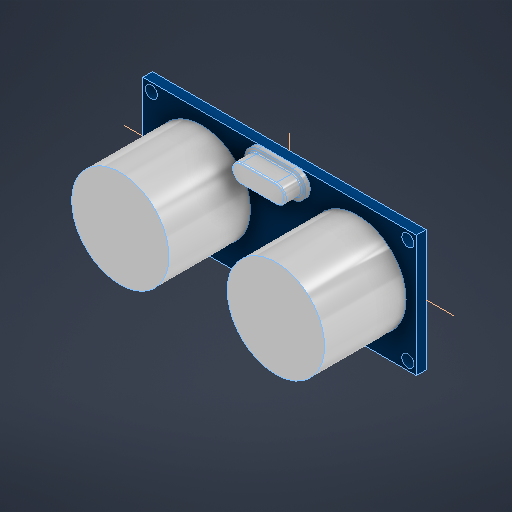
# Autodesk Inventor part: ultrasonic-sensor-2-group2
Saved by Autodesk Inventor 2026.2 (Build 302298010, 298A)
## iProperties
Created: 2026-02-24
Part Number: ultrasonic-sensor-2-group2
Material: Generic
Document SubType Name: Modeling
Designer: ts2104
Density: 1 g/cm^3
Appearance: Default
Author: ts2104
Autodesk Inventor part; units mm, degrees
ref_plane "YZ Plane" through (0, 0, 0) normal (1, 0, 0) x (0, 1, 0)
sketch "Sketch1" plane through (0, 0, 0) normal (0, 0, 1) x (1, 0, 0)
  line L0 (-22.5, 10) -> (22.5, 10)
  line L1 (22.5, 10) -> (22.5, -10)
  line L2 (22.5, -10) -> (-22.5, -10)
  line L3 (-22.5, -10) -> (-22.5, 10)
  line L4 (-22.5, 10) -> (22.5, -10) construction
  line L5 (22.5, 10) -> (-22.5, -10) construction
  line L6 (-31.5, 0) -> (31.5, 0) projected
  line L7 (0, -14) -> (0, 14) projected
  circle A0 centre (-12.8, 0) radius 8
  circle A1 centre (-21.1, -8.6) radius 1
  circle A2 centre (-21.1, 8.6) radius 1
  circle A3 centre (12.8, 0) radius 8
  circle A4 centre (21.1, -8.6) radius 1
  circle A5 centre (21.1, 8.6) radius 1
  line L8 (-5.08, -6.96) -> (5.08, -6.96)
  line L9 (5.08, -6.96) -> (5.08, -9.5)
  line L10 (5.08, -9.5) -> (-5.08, -9.5)
  line L11 (-5.08, -9.5) -> (-5.08, -6.96)
  line L12 (-5.08, -6.96) -> (5.08, -9.5) construction
  line L13 (5.08, -6.96) -> (-5.08, -9.5) construction
  line L14 (-4.13, -7.91) -> (-3.49, -7.91)
  line L15 (-3.49, -7.91) -> (-3.49, -8.55)
  line L16 (-3.49, -8.55) -> (-4.13, -8.55)
  line L17 (-4.13, -8.55) -> (-4.13, -7.91)
  line L18 (-4.13, -7.91) -> (-3.49, -8.55) construction
  line L19 (-3.49, -7.91) -> (-4.13, -8.55) construction
  line L20 (-5.08, -8.23) -> (5.08, -8.23)
  line L21 (-0.95, -7.91) -> (-1.59, -8.55) construction
  line L22 (-1.59, -7.91) -> (-0.95, -8.55) construction
  line L23 (-0.95, -8.55) -> (-1.59, -8.55)
  line L24 (-1.59, -7.91) -> (-0.95, -7.91)
  line L25 (-0.95, -7.91) -> (-0.95, -8.55)
  line L26 (-1.59, -8.55) -> (-1.59, -7.91)
  line L27 (1.59, -7.91) -> (0.95, -8.55) construction
  line L28 (0.95, -7.91) -> (1.59, -8.55) construction
  line L29 (1.59, -8.55) -> (0.95, -8.55)
  line L30 (0.95, -7.91) -> (1.59, -7.91)
  line L31 (1.59, -7.91) -> (1.59, -8.55)
  line L32 (0.95, -8.55) -> (0.95, -7.91)
  line L33 (4.13, -7.91) -> (3.49, -8.55) construction
  line L34 (3.49, -7.91) -> (4.13, -8.55) construction
  line L35 (4.13, -8.55) -> (3.49, -8.55)
  line L36 (3.49, -7.91) -> (4.13, -7.91)
  line L37 (4.13, -7.91) -> (4.13, -8.55)
  line L38 (3.49, -8.55) -> (3.49, -7.91)
  line L39 (-2.85, 10) -> (2.85, 10)
  line L40 (2.85, 10) -> (2.85, 5.6)
  line L41 (2.85, 5.6) -> (-2.85, 5.6)
  line L42 (-2.85, 5.6) -> (-2.85, 10)
  line L43 (-2.85, 10) -> (2.85, 5.6) construction
  line L44 (2.85, 10) -> (-2.85, 5.6) construction
  circle A6 centre (-2.85, 7.8) radius 2.2
  circle A7 centre (2.85, 7.8) radius 2.2
  circle A8 centre (-2.85, 7.8) radius 1.55
  line L45 (-2.85, 9.35) -> (2.85, 9.35)
  line L46 (2.85, 9.35) -> (2.85, 6.25)
  line L47 (2.85, 6.25) -> (-2.85, 6.25)
  line L48 (-2.85, 6.25) -> (-2.85, 9.35)
  line L49 (-2.85, 9.35) -> (2.85, 6.25) construction
  line L50 (2.85, 9.35) -> (-2.85, 6.25) construction
  circle A9 centre (2.85, 7.8) radius 1.55
  point P0 (0, 0)
  point P1 (0, -8.23)
  point P2 (-3.81, -8.23)
  point P3 (-1.27, -8.23)
  point P4 (1.27, -8.23)
  point P5 (3.81, -8.23)
  point P6 (0, 7.8)
  point P7 (2.85, 9.35)
  point P8 (-2.85, 6.25)
  dimension "d0" = 45
  dimension "d1" = 20
  dimension "d3" = 16
  dimension "d4" = 1.4
  dimension "d5" = 1.4
  dimension "d9" = 2
  dimension "d10" = 10.16
  dimension "d11" = 2.54
  dimension "d12" = 0.5
  dimension "d13" = 0.64
  dimension "d15" = 1.27
  dimension "d18" = 2.54
  dimension "d46" = 12.8
  dimension "d47" = 4.4
  dimension "d49" = 5.7
  dimension "d52" = 3.1
  constraints: 98 end point, 13 midpoint, 10 parallel, 8 centre point, 6 horizontal, 6 perpendicular, 6 symmetric about line, 5 point on line, 1 coincident, 1 collinear, 47 other
  measures "d0" distance of L0.start L0.end
  measures "d1" distance of L2.end L0.start
  measures "d3" diameter of A0
  measures "d4" distance from line of L3 A1.centre
  measures "d5" distance from line of A1.centre L2
  measures "d9" diameter of A1
  measures "d10" distance of L9.end L10.end
  measures "d11" distance between parallel lines of L10 L8
  measures "d12" distance between parallel lines of L2 L10
  measures "d13" distance of L16.end L14.start
  measures "d15" distance from line of L11 point (-3.81, -8.23)
  measures "d18" distance of L14.end L21.start
  measures "d46" distance from line of L7 A0.centre
  measures "d47" distance of L39.end L40.end
  measures "d49" distance of L39.start L39.end
  measures "d52" distance between parallel lines of L47 L45
extrude "Extrusion1" add sketch "Sketch1" along normal blind 1.6 contours L0 A6 L41 L7 L6 A0 L3 | A6 L45 L42 | L42 A8 A6 | L0 L7 L45 A6 | L6 A0 L7 L8 L11 L10 L2 L3 | L0 A7 L45 L7 | A8 L42 | L45 A6 L47 A8 | L42 A8 | A6 L47 L7 L41 | L42 L47 A6 | L45 L7 L47 A6 | A0 L6 | L6 A0 | A7 L40 A9 | L0 L1 L6 A3 L7 L41 A7 | L40 L45 A7 | L45 A7 L47 L7 | L7 L47 A7 L41 | L7 L10 L9 L8 L6 A3 L1 L2 | A9 L40 | A9 L47 A7 L45 | L40 A9 | A7 L47 L40 | L10 L11 L20 L17 L16 L15 L26 L23 L25 L7 | L7 L20 L32 L29 L31 L38 L35 L37 L9 L10 | A3 L6 | L6 A3 | L8 L9 L20 L37 L36 L38 L31 L30 L32 L7 | L7 L20 L25 L24 L26 L15 L14 L17 L11 L8
extrude "Extrusion2" add sketch "Sketch1" along normal blind 15 contours A0 L6 | L6 A0 | A3 L6 | L6 A3
extrude "Extrusion3" add sketch "Sketch1" against normal blind 2.4 contours L10 L11 L20 L17 L16 L15 L26 L23 L25 L7 | L7 L20 L32 L29 L31 L38 L35 L37 L9 L10 | L8 L9 L20 L37 L36 L38 L31 L30 L32 L7 | L7 L20 L25 L24 L26 L15 L14 L17 L11 L8
extrude "Extrusion4" add sketch "Sketch1" along normal blind 3 and the other way blind 3.4 separate body contours L25 L23 L26 L20 | L20 L26 L24 L25 | L32 L30 L31 L20 | L20 L31 L29 L32 | L37 L35 L38 L20 | L20 L38 L36 L37 | L20 L15 L16 L17 | L17 L14 L15 L20
sketch "Sketch2" plane through (0, 0, -3.4) normal (0, 0, -1) x (-1, 0, 0)
  line L0 (-4.13, -7.91) -> (-4.13, -8.55) projected
  line L1 (-4.13, -8.55) -> (-3.49, -8.55) projected
  line L2 (-3.49, -8.55) -> (-3.49, -7.91) projected
  line L3 (-3.49, -7.91) -> (-4.13, -7.91) projected
  line L4 (-1.59, -7.91) -> (-1.59, -8.55) projected
  line L5 (-1.59, -8.55) -> (-0.95, -8.55) projected
  line L6 (-0.95, -8.55) -> (-0.95, -7.91) projected
  line L7 (-0.95, -7.91) -> (-1.59, -7.91) projected
  line L8 (0.95, -7.91) -> (0.95, -8.55) projected
  line L9 (0.95, -8.55) -> (1.59, -8.55) projected
  line L10 (1.59, -8.55) -> (1.59, -7.91) projected
  line L11 (1.59, -7.91) -> (0.95, -7.91) projected
  line L12 (3.49, -7.91) -> (3.49, -8.55) projected
  line L13 (3.49, -8.55) -> (4.13, -8.55) projected
  line L14 (4.13, -8.55) -> (4.13, -7.91) projected
  line L15 (4.13, -7.91) -> (3.49, -7.91) projected
  point P0 (0, 0)
revolve "Revolution1" add sketch "Sketch2" angle 90 about axis through (4.13, -8.55, -3.4) along (-1, 0, 0) bodies 2
sketch "Sketch3" plane through (0.95, -8.55, 3) normal (0, -1, 0) x (1, 0, 0)
  line L0 (0, -6.4) -> (0.64, -6.4) projected
  line L1 (2.54, -6.4) -> (3.18, -6.4) projected
  line L2 (-2.54, -6.4) -> (-1.9, -6.4) projected
  line L3 (-5.08, -6.4) -> (-4.44, -6.4) projected
  line L4 (-5.08, -7.04) -> (-5.08, 0) projected
  line L5 (-5.08, -7.04) -> (-4.44, -7.04)
  line L6 (-4.44, -7.04) -> (-4.44, -6.4)
  line L7 (-4.44, -6.4) -> (-5.08, -6.4)
  line L8 (-5.08, -6.4) -> (-5.08, -7.04)
  line L9 (-2.54, -7.04) -> (-1.9, -7.04)
  line L10 (-1.9, -7.04) -> (-1.9, -6.4)
  line L11 (-1.9, -6.4) -> (-2.54, -6.4)
  line L12 (-2.54, -6.4) -> (-2.54, -7.04)
  line L13 (0, -7.04) -> (0.64, -7.04)
  line L14 (0.64, -7.04) -> (0.64, -6.4)
  line L15 (0.64, -6.4) -> (0, -6.4)
  line L16 (0, -6.4) -> (0, -7.04)
  line L17 (2.54, -7.04) -> (3.18, -7.04)
  line L18 (3.18, -7.04) -> (3.18, -6.4)
  line L19 (3.18, -6.4) -> (2.54, -6.4)
  line L20 (2.54, -6.4) -> (2.54, -7.04)
  point P0 (-0.95, -3)
  dimension "d36" = 2.54
  constraints: 32 end point, 2 horizontal, 2 parallel, 1 perpendicular, 27 other
  measures "d36" distance of L3.start point (-2.54, -6.4)
extrude "Extrusion5" add sketch "Sketch3" along normal blind 6 separate body
sketch "Sketch4" plane through (0, 0, 1.6) normal (0, 0, 1) x (1, 0, 0)
  circle A0 centre (-12.8, 0) radius 8 projected
  circle A1 centre (12.8, 0) radius 8 projected
  point P0 (0, 0)
combine bodies "Combine1" operation type add bodies to combine 3 2
ref_plane "Work Plane1" through (0, 0, 1.6) normal (0, 0, 1) x (1, 0, 0)
split body "Split1" result two bodies by plane through (0, 0, 1.6) normal (0, 0, 1) bodies 1 first body at (-5.3971, 1.2031, 6.0667) (20.2029, 1.2031, 6.0667)
fillet "Fillet1" radius 0.2 4 edges at (-3.81, -8.55, -3.4) (-1.27, -8.55, -3.4) (1.27, -8.55, -3.4) (3.81, -8.55, -3.4)
combine bodies "Combine2" operation type add bodies to combine 5 4 3
fillet "Fillet2" radius 0.75 16 edges at (-3.81, -8.55, 1.6) (-3.49, -8.23, 1.6) (-4.13, -8.23, 1.6) (-3.81, -7.91, 1.6) (-1.27, -8.55, 1.6) (-1.59, -8.23, 1.6) (-1.27, -7.91, 1.6) (-0.95, -8.23, 1.6) (1.59, -8.23, 1.6) (1.27, -8.55, 1.6) (0.95, -8.23, 1.6) (1.27, -7.91, 1.6) (3.49, -8.23, 1.6) (3.81, -8.55, 1.6) (4.13, -8.23, 1.6) (3.81, -7.91, 1.6)
extrude "Extrusion6" add sketch "Sketch1" along normal blind 2.3 contours A6 L45 L42 | L42 A8 A6 | L0 L7 L45 A6 | L0 A7 L45 L7 | A8 L42 | L45 A6 L47 A8 | L42 A8 | A6 L47 L7 L41 | L42 L47 A6 | L45 L7 L47 A6 | A7 L40 A9 | L40 L45 A7 | L45 A7 L47 L7 | L7 L47 A7 L41 | A9 L40 | A9 L47 A7 L45 | L40 A9 | A7 L47 L40 bodies 5
extrude "Extrusion7" add sketch "Sketch1" along normal blind 5.1 contours A8 L42 | L45 A6 L47 A8 | L42 A8 | L45 L7 L47 A6 | L45 A7 L47 L7 | A9 L40 | A9 L47 A7 L45 | L40 A9 bodies 5
ref_plane "Work Plane2" through (0, 0, 1.6) normal (0, 0, 1) x (1, 0, 0)
split_face "Split2"
fillet "Fillet3" radius 0.2 4 edges at (-4.4, 7.8, 2.3) (0, 9.35, 2.3) (4.4, 7.8, 2.3) (0, 6.25, 2.3)
fillet "Fillet4" radius 0.2 4 edges at (-4.4, 7.8, 5.1) (0, 6.25, 5.1) (4.4, 7.8, 5.1) (0, 9.35, 5.1)
equation "\"d5\" = d4"
equation "\"d10\" = 4 * d11"
equation "\"d15\" = 0.5 * d11"
equation "\"d18\" = d11"
